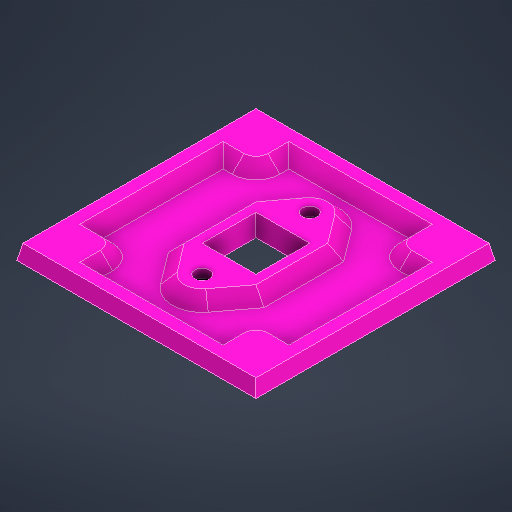
# Autodesk Inventor part: Camera Cover
Saved by Autodesk Inventor 2025.1 (Build 291241000, 241)
## iProperties
Created: 2024-11-09
Part Number: Camera Cover
Material: Generic
Document SubType Name: Modeling
Designer: jerem
Density: 1 g/cm^3
Appearance: Default
Author: jerem
## iProperties of the stored document Camera Cover_3DPrint.ipt
Created: 2024-11-09
Part Number: Camera Cover_3DPrint
Material: Generic
Document SubType Name: Modeling
Designer: jerem
Density: 1 g/cm^3
Appearance: Default
Author: jerem
Autodesk Inventor part; units mm, degrees
ref_plane "YZ Plane" through (0, 0, 0) normal (1, 0, 0) x (0, 1, 0)
ref_plane "XZ Plane" through (0, 0, 0) normal (0, 1, 0) x (-1, 0, 0)
ref_plane "XY Plane" through (0, 0, 0) normal (0, 0, 1) x (1, 0, 0)
sketch "Sketch1" plane through (0, 0, 0) normal (0, 1, 0) x (-1, 0, 0)
  line L0 (-20, -20) -> (20, -20)
  line L1 (20, -20) -> (20, 20)
  line L2 (20, 20) -> (-20, 20)
  line L3 (-20, 20) -> (-20, -20)
  line L4 (-20, -20) -> (20, 20) construction
  line L5 (20, -20) -> (-20, 20) construction
  line L6 (-4.5, -4.5) -> (4.5, -4.5)
  line L7 (4.5, -4.5) -> (4.5, 4.5)
  line L8 (4.5, 4.5) -> (-4.5, 4.5)
  line L9 (-4.5, 4.5) -> (-4.5, -4.5)
  line L10 (-4.5, -4.5) -> (4.5, 4.5) construction
  line L11 (4.5, -4.5) -> (-4.5, 4.5) construction
  circle A0 centre (0, -9) radius 1.25
  line L12 (0, -9) -> (0, 0) construction
  circle A1 centre (0, -9) radius 2
  circle A2 centre (0, 9) radius 2
  line L13 (0, 9) -> (0, 0) construction
  circle A3 centre (0, 9) radius 1.25
  circle A4 centre (14, 14) radius 2
  circle A5 centre (-14, 14) radius 2
  circle A6 centre (-14, -14) radius 2
  circle A7 centre (14, -14) radius 2
  line L14 (14, 14) -> (14, -14) construction
  line L15 (14, 14) -> (-14, 14) construction
  line L16 (-14, -14) -> (-14, 14) construction
  circle A8 centre (-14, -14) radius 1.3
  circle A9 centre (-14, 14) radius 1.3
  circle A10 centre (14, 14) radius 1.3
  circle A11 centre (14, -14) radius 1.3
  circle A12 centre (0, -9) radius 3
  circle A13 centre (0, 9) radius 3
  line L17 (-17.5, -17.5) -> (17.5, -17.5)
  line L18 (17.5, -17.5) -> (17.5, 17.5)
  line L19 (17.5, 17.5) -> (-17.5, 17.5)
  line L20 (-17.5, 17.5) -> (-17.5, -17.5)
  line L21 (-6, -6) -> (6, -6)
  line L22 (6, -6) -> (6, 6)
  line L23 (6, 6) -> (-6, 6)
  line L24 (-6, 6) -> (-6, -6)
  line L25 (-6, 6) -> (-2.4, 10.8)
  line L26 (2.4, 10.8) -> (6, 6)
  line L27 (6, -6) -> (2.4, -10.8)
  line L28 (-2.4, -10.8) -> (-6, -6)
  line L29 (14, -12) -> (17.5, -12)
  line L30 (12, -14) -> (12, -17.5)
  line L31 (17.5, 12) -> (14, 12)
  line L32 (12, 14) -> (12, 17.5)
  line L33 (-12, 14) -> (-12, 17.5)
  line L34 (-14, 12) -> (-17.5, 12)
  line L35 (-14, -12) -> (-17.5, -12)
  line L36 (-12, -14) -> (-12, -17.5)
  point P0 (0, -6)
  point P1 (0, 6)
  dimension "d0" = 40
  dimension "d2" = 9
  dimension "d3" = 2.5
  dimension "d4" = 9
  dimension "d5" = 4
  dimension "d16" = 4
  dimension "d17" = 28
  dimension "d27" = 2.6
  dimension "d45" = 6
  dimension "d48" = 1.5
  dimension "d49" = 2.5
  constraints: 74 end point, 27 point on line, 14 centre point, 12 point on circle, 9 equal radius, 8 coincident, 8 parallel, 8 perpendicular, 8 tangent, 4 midpoint, 4 vertical, 2 equal length, 2 horizontal, 3 other
  measures "d0" distance of L1.end L2.end
  measures "d2" distance of L6.end L7.end
  measures "d3" diameter of A0
  measures "d4" distance of L12.end L12.start
  measures "d5" diameter of A1
  measures "d16" diameter of A4
  measures "d17" distance of L14.start L15.end
  measures "d27" diameter of A8
  measures "d45" diameter of A12
  measures "d48" distance between parallel lines of L9 L24
  measures "d49" distance between parallel lines of L0 L17
extrude "Extrusion1" add sketch "Sketch1" against normal blind 1.7 contours L3 L2 L1 L0 | A1 | A2 | A4 | A4 L32 L19 L18 L31 | A4 L31 L18 L29 A7 L30 L17 L36 A6 L35 L20 L34 A5 L33 L19 L32 | L33 A5 L34 L20 L19 | L18 L17 L30 A7 L29 | A5 | A7 | L35 A6 L36 L17 L20 | A6 | A8 | A9 | A10 | A11 | A12 | L28 L21 A12 | A12 L21 L27 | L21 L24 L23 L22 | L25 A13 L23 | L23 A13 L26 | A13
extrude "Extrusion3" add sketch "Sketch1" along normal blind 2 contours L3 L2 L1 L0 | A1 | A2 | A4 | A4 L32 L19 L18 L31 | L33 A5 L34 L20 L19 | L18 L17 L30 A7 L29 | A5 | A7 | L35 A6 L36 L17 L20 | A6 | A8 | A9 | A10 | A11 | A12 | L28 L21 A12 | A12 L21 L27 | L21 L24 L23 L22 | L25 A13 L23 | L23 A13 L26 | A13
extrude "Extrusion2" cut sketch "Sketch1" along normal blind 2.2 from surface at -1.7 contours A1 | A2
chamfer "Chamfer7" distance 2 angle 45 24 edges at (0, 0, -17.5) (17.5, 0, 0) (12.5858, 0, -12.5858) (12, 0, -15.75) (15.75, 0, -12) (12, 0, 15.75) (12.5858, 0, 12.5858) (15.75, 0, 12) (0, 0, 17.5) (-12.5858, 0, 12.5858) (-12, 0, 15.75) (-15.75, 0, 12) (-17.5, 0, 0) (-12, 0, -15.75) (-12.5858, 0, -12.5858) (-15.75, 0, -12) (-4.2, 0, -8.4) (0, 0, -12) (4.2, 0, -8.4) (-6, 0, 0) (-4.2, 0, 8.4) (0, 0, 12) (4.2, 0, 8.4) (6, 0, 0)
chamfer "Chamfer8" distance 0.5 distance2 2.5 4 edges at (0, 2, -20) (-20, 2, 0) (20, 2, 0) (0, 2, 20) measured on face at (19.5, 2, 0) measured on face at (-19.5, 2, 0) measured on face at (0, 2, -19.5) measured on face at (0, 2, 19.5)
chamfer "Chamfer9" distance 3 distance2 1.2 4 edges at (0, -1.7, -20) (20, -1.7, 0) (0, -1.7, 20) (-20, -1.7, 0) measured on face at (0, -1.7, -19.5) measured on face at (-19.5, -1.7, 0) measured on face at (19.5, -1.7, 0) measured on face at (0, -1.7, 19.5)
body "Solid1"
